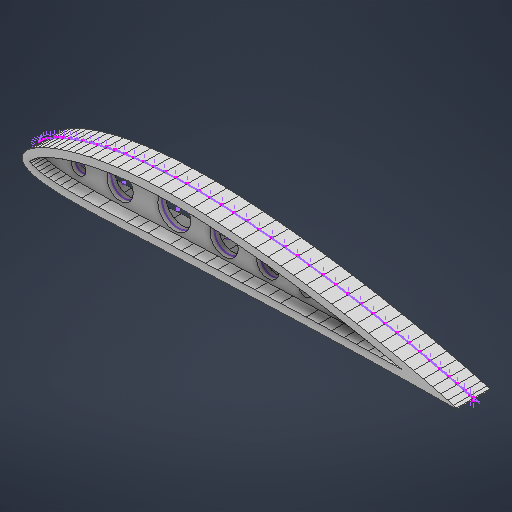
# Autodesk Inventor part: Profil NACA 4412
Saved by Autodesk Inventor 2026 (Build 300175050, 175E)
## iProperties
Created: 2026-01-17
Part Number: Profil NACA 4412
Material: Všeobecné
Document SubType Name: Modeling
Designer: marti
Density: 1 g/cm^3
Appearance: Výchozí
Author: marti
Autodesk Inventor part; units mm, degrees
ref_plane "YZ Plane" through (0, 0, 0) normal (1, 0, 0) x (0, 1, 0)
ref_plane "XZ Plane" through (0, 0, 0) normal (0, 1, 0) x (-1, 0, 0)
ref_plane "XY Plane" through (0, 0, 0) normal (0, 0, 1) x (1, 0, 0)
sketch "Náčrt1" plane through (-64.9965, -4.5129, 0) normal (0, 0, 1) x (1, 0, 0)
  line L0 (0, 0) -> (0.1008, -0.6172)
  line L1 (0.1008, -0.6172) -> (0.4005, -1.1751)
  line L2 (0.4005, -1.1751) -> (0.8948, -1.675)
  line L3 (0.8948, -1.675) -> (1.5794, -2.1181)
  line L4 (1.5794, -2.1181) -> (2.45, -2.5059)
  line L5 (2.45, -2.5059) -> (3.502, -2.8399)
  line L6 (3.502, -2.8399) -> (4.7309, -3.1217)
  line L7 (4.7309, -3.1217) -> (6.1321, -3.3532)
  line L8 (6.1321, -3.3532) -> (7.7009, -3.5364)
  line L9 (7.7009, -3.5364) -> (9.4326, -3.6734)
  line L10 (9.4326, -3.6734) -> (11.3221, -3.7667)
  line L11 (11.3221, -3.7667) -> (13.3646, -3.8188)
  line L12 (13.3646, -3.8188) -> (15.5549, -3.8188)
  line L13 (15.5549, -3.8188) -> (17.8877, -3.8188)
  line L14 (17.8877, -3.8188) -> (20.3578, -3.7585)
  line L15 (20.3578, -3.7585) -> (22.9603, -3.695)
  line L16 (22.9603, -3.695) -> (25.688, -3.5719)
  line L17 (25.688, -3.5719) -> (28.5365, -3.4433)
  line L18 (28.5365, -3.4433) -> (31.5001, -3.3096)
  line L19 (31.5001, -3.3096) -> (34.5717, -3.1509)
  line L20 (34.5717, -3.1509) -> (37.7458, -2.9903)
  line L21 (37.7458, -2.9903) -> (41.0158, -2.8272)
  line L22 (41.0158, -2.8272) -> (44.3749, -2.6597)
  line L23 (44.3749, -2.6597) -> (47.817, -2.512)
  line L24 (47.817, -2.512) -> (51.3342, -2.369)
  line L25 (51.3342, -2.369) -> (54.9194, -2.2327)
  line L26 (54.9194, -2.2327) -> (58.5651, -2.0885)
  line L27 (58.5651, -2.0885) -> (62.2634, -1.9385)
  line L28 (62.2634, -1.9385) -> (66.0059, -1.7856)
  line L29 (66.0059, -1.7856) -> (69.7841, -1.632)
  line L30 (69.7841, -1.632) -> (73.5888, -1.4803)
  line L31 (73.5888, -1.4803) -> (77.4106, -1.3325)
  line L32 (77.4106, -1.3325) -> (85.0644, -1.0556)
  line L33 (85.0644, -1.0556) -> (88.8745, -0.9296)
  line L34 (88.8745, -0.9296) -> (92.6573, -0.8132)
  line L35 (92.6573, -0.8132) -> (96.3998, -0.7072)
  line L36 (96.3998, -0.7072) -> (100.0878, -0.612)
  line L37 (100.0878, -0.612) -> (103.7057, -0.5276)
  line L38 (103.7057, -0.5276) -> (107.2363, -0.4539)
  line L39 (107.2363, -0.4539) -> (110.6603, -0.3905)
  line L40 (110.6603, -0.3905) -> (113.9558, -0.3368)
  line L41 (113.9558, -0.3368) -> (117.0974, -0.2918)
  line L42 (117.0974, -0.2918) -> (120.055, -0.2549)
  line L43 (120.055, -0.2549) -> (122.7911, -0.2251)
  line L44 (122.7911, -0.2251) -> (125.2574, -0.2014)
  line L45 (125.2574, -0.2014) -> (127.3856, -0.1834)
  line L46 (127.3856, -0.1834) -> (129.0641, -0.1691)
  line L47 (129.0641, -0.1691) -> (129.9931, -0.1612)
  line L48 (129.9931, -0.1612) -> (129.9906, 0.1321)
  line L49 (129.9906, 0.1321) -> (129.0576, 0.3875)
  line L50 (129.0576, 0.3875) -> (127.3795, 0.839)
  line L51 (127.3795, 0.839) -> (125.2516, 1.3993)
  line L52 (125.2516, 1.3993) -> (122.7858, 2.032)
  line L53 (122.7858, 2.032) -> (120.0501, 2.7132)
  line L54 (120.0501, 2.7132) -> (117.0931, 3.4254)
  line L55 (117.0931, 3.4254) -> (113.952, 4.1548)
  line L56 (113.952, 4.1548) -> (110.657, 4.8904)
  line L57 (110.657, 4.8904) -> (107.2335, 5.6228)
  line L58 (107.2335, 5.6228) -> (103.7034, 6.3444)
  line L59 (103.7034, 6.3444) -> (100.086, 7.0485)
  line L60 (100.086, 7.0485) -> (96.3985, 7.7294)
  line L61 (96.3985, 7.7294) -> (92.6565, 8.3822)
  line L62 (92.6565, 8.3822) -> (88.8741, 9.0026)
  line L63 (88.8741, 9.0026) -> (85.0644, 9.5868)
  line L64 (85.0644, 9.5868) -> (81.2394, 10.1289)
  line L65 (81.2394, 10.1289) -> (77.4106, 10.6287)
  line L66 (77.4106, 10.6287) -> (73.5888, 11.0836)
  line L67 (73.5888, 11.0836) -> (69.7841, 11.4914)
  line L68 (69.7841, 11.4914) -> (66.0059, 11.8502)
  line L69 (66.0059, 11.8502) -> (62.2634, 12.1585)
  line L70 (62.2634, 12.1585) -> (58.5651, 12.4148)
  line L71 (58.5651, 12.4148) -> (54.9194, 12.6181)
  line L72 (54.9194, 12.6181) -> (51.3342, 12.7673)
  line L73 (51.3342, 12.7673) -> (47.817, 12.8447)
  line L74 (47.817, 12.8447) -> (44.3752, 12.8426)
  line L75 (44.3752, 12.8426) -> (41.0158, 12.7632)
  line L76 (41.0158, 12.7632) -> (37.7458, 12.6088)
  line L77 (37.7458, 12.6088) -> (34.5717, 12.3826)
  line L78 (34.5717, 12.3826) -> (31.4999, 12.088)
  line L79 (31.4999, 12.088) -> (28.5366, 11.7287)
  line L80 (28.5366, 11.7287) -> (25.688, 11.3091)
  line L81 (25.688, 11.3091) -> (22.9598, 10.8338)
  line L82 (22.9598, 10.8338) -> (20.3578, 10.3077)
  line L83 (20.3578, 10.3077) -> (17.8877, 9.7359)
  line L84 (17.8877, 9.7359) -> (15.5548, 9.1241)
  line L85 (15.5548, 9.1241) -> (13.3646, 8.4777)
  line L86 (13.3646, 8.4777) -> (11.3221, 7.8025)
  line L87 (11.3221, 7.8025) -> (9.4326, 7.1042)
  line L88 (9.4326, 7.1042) -> (7.7009, 6.3887)
  line L89 (7.7009, 6.3887) -> (6.1321, 5.6614)
  line L90 (6.1321, 5.6614) -> (4.7309, 4.928)
  line L91 (4.7309, 4.928) -> (3.502, 4.1935)
  line L92 (3.502, 4.1935) -> (2.45, 3.4628)
  line L93 (2.45, 3.4628) -> (1.5794, 2.7403)
  line L94 (1.5794, 2.7403) -> (0.8948, 2.0298)
  line L95 (0.8948, 2.0298) -> (0.4005, 1.3347)
  line L96 (0.4005, 1.3347) -> (0.1008, 0.6574)
  line L97 (0.1008, 0.6574) -> (0, 0)
  point P0 (81.2394, -1.1904)
  constraints: 196 end point, 7 collinear, 2 perpendicular, 1 horizontal, 1 parallel
sketch "Náčrt2" plane through (0, 0, 0) normal (0, 0, 1) x (1, 0, 0)
  line L0 (-64.8957, -5.1301) -> (-64.596, -5.688) projected
  line L1 (-64.596, -5.688) -> (-64.1017, -6.1879) projected
  line L2 (-64.1017, -6.1879) -> (-63.4171, -6.631) projected
  line L3 (-63.4171, -6.631) -> (-62.5466, -7.0188) projected
  line L4 (-62.5466, -7.0188) -> (-61.4946, -7.3528) projected
  line L5 (-61.4946, -7.3528) -> (-60.2657, -7.6347) projected
  line L6 (-60.2657, -7.6347) -> (-58.8644, -7.8662) projected
  line L7 (-58.8644, -7.8662) -> (-57.2956, -8.0493) projected
  line L8 (-57.2956, -8.0493) -> (-55.564, -8.1863) projected
  line L9 (-55.564, -8.1863) -> (-53.6744, -8.2796) projected
  line L10 (-53.6744, -8.2796) -> (-51.632, -8.3318) projected
  line L11 (-51.632, -8.3318) -> (-47.1088, -8.3318) projected
  line L12 (-47.1088, -8.3318) -> (-42.0363, -8.208) projected
  line L13 (-42.0363, -8.208) -> (-33.4964, -7.8225) projected
  line L14 (-33.4964, -7.8225) -> (-30.4248, -7.6638) projected
  line L15 (-30.4248, -7.6638) -> (-27.2507, -7.5032) projected
  line L16 (-27.2507, -7.5032) -> (-20.6217, -7.1726) projected
  line L17 (-20.6217, -7.1726) -> (-17.1795, -7.0249) projected
  line L18 (-17.1795, -7.0249) -> (-13.6624, -6.882) projected
  line L19 (-13.6624, -6.882) -> (-10.0771, -6.7456) projected
  line L20 (-10.0771, -6.7456) -> (-6.4314, -6.6014) projected
  line L21 (-6.4314, -6.6014) -> (-2.7331, -6.4515) projected
  line L22 (-2.7331, -6.4515) -> (1.0094, -6.2985) projected
  line L23 (1.0094, -6.2985) -> (4.7875, -6.1449) projected
  line L24 (4.7875, -6.1449) -> (8.5923, -5.9932) projected
  line L25 (8.5923, -5.9932) -> (12.4141, -5.8454) projected
  line L26 (12.4141, -5.8454) -> (20.0679, -5.5686) projected
  line L27 (20.0679, -5.5686) -> (23.878, -5.4425) projected
  line L28 (23.878, -5.4425) -> (27.6608, -5.3262) projected
  line L29 (27.6608, -5.3262) -> (31.4033, -5.2202) projected
  line L30 (31.4033, -5.2202) -> (35.0913, -5.1249) projected
  line L31 (35.0913, -5.1249) -> (38.7092, -5.0406) projected
  line L32 (38.7092, -5.0406) -> (42.2397, -4.9669) projected
  line L33 (42.2397, -4.9669) -> (45.6637, -4.9035) projected
  line L34 (45.6637, -4.9035) -> (48.9593, -4.8497) projected
  line L35 (48.9593, -4.8497) -> (52.1009, -4.8048) projected
  line L36 (52.1009, -4.8048) -> (55.0584, -4.7678) projected
  line L37 (55.0584, -4.7678) -> (57.7946, -4.738) projected
  line L38 (57.7946, -4.738) -> (60.2609, -4.7144) projected
  line L39 (60.2609, -4.7144) -> (64.9965, -4.6742) projected
  line L40 (64.9965, -4.6742) -> (64.994, -4.3808) projected
  line L41 (64.994, -4.3808) -> (64.0611, -4.1254) projected
  line L42 (64.0611, -4.1254) -> (62.3829, -3.6739) projected
  line L43 (62.3829, -3.6739) -> (60.2551, -3.1136) projected
  line L44 (60.2551, -3.1136) -> (57.7893, -2.481) projected
  line L45 (57.7893, -2.481) -> (55.0536, -1.7998) projected
  line L46 (55.0536, -1.7998) -> (52.0966, -1.0876) projected
  line L47 (52.0966, -1.0876) -> (48.9554, -0.3581) projected
  line L48 (48.9554, -0.3581) -> (45.6604, 0.3774) projected
  line L49 (45.6604, 0.3774) -> (42.237, 1.1099) projected
  line L50 (42.237, 1.1099) -> (38.7069, 1.8315) projected
  line L51 (38.7069, 1.8315) -> (35.0895, 2.5356) projected
  line L52 (35.0895, 2.5356) -> (31.402, 3.2165) projected
  line L53 (31.402, 3.2165) -> (27.66, 3.8692) projected
  line L54 (27.66, 3.8692) -> (23.8776, 4.4896) projected
  line L55 (23.8776, 4.4896) -> (20.0679, 5.0739) projected
  line L56 (20.0679, 5.0739) -> (16.2428, 5.616) projected
  line L57 (16.2428, 5.616) -> (12.4141, 6.1158) projected
  line L58 (12.4141, 6.1158) -> (8.5923, 6.5707) projected
  line L59 (8.5923, 6.5707) -> (4.7875, 6.9785) projected
  line L60 (4.7875, 6.9785) -> (1.0094, 7.3373) projected
  line L61 (1.0094, 7.3373) -> (-2.7331, 7.6455) projected
  line L62 (-2.7331, 7.6455) -> (-6.4314, 7.9018) projected
  line L63 (-6.4314, 7.9018) -> (-10.0771, 8.1052) projected
  line L64 (-10.0771, 8.1052) -> (-13.6624, 8.2544) projected
  line L65 (-13.6624, 8.2544) -> (-17.1795, 8.3318) projected
  line L66 (-17.1795, 8.3318) -> (-20.6213, 8.3297) projected
  line L67 (-20.6213, 8.3297) -> (-23.9807, 8.2502) projected
  line L68 (-23.9807, 8.2502) -> (-27.2507, 8.0959) projected
  line L69 (-27.2507, 8.0959) -> (-30.4248, 7.8697) projected
  line L70 (-30.4248, 7.8697) -> (-33.4966, 7.575) projected
  line L71 (-33.4966, 7.575) -> (-36.4599, 7.2158) projected
  line L72 (-36.4599, 7.2158) -> (-39.3086, 6.7962) projected
  line L73 (-39.3086, 6.7962) -> (-42.0367, 6.3209) projected
  line L74 (-42.0367, 6.3209) -> (-44.6387, 5.7947) projected
  line L75 (-44.6387, 5.7947) -> (-47.1088, 5.223) projected
  line L76 (-47.1088, 5.223) -> (-49.4417, 4.6111) projected
  line L77 (-49.4417, 4.6111) -> (-51.632, 3.9647) projected
  line L78 (-51.632, 3.9647) -> (-53.6744, 3.2895) projected
  line L79 (-53.6744, 3.2895) -> (-55.564, 2.5913) projected
  line L80 (-55.564, 2.5913) -> (-57.2956, 1.8757) projected
  line L81 (-57.2956, 1.8757) -> (-58.8644, 1.1485) projected
  line L82 (-58.8644, 1.1485) -> (-60.2657, 0.4151) projected
  line L83 (-60.2657, 0.4151) -> (-61.4946, -0.3194) projected
  line L84 (-61.4946, -0.3194) -> (-62.5466, -1.0501) projected
  line L85 (-62.5466, -1.0501) -> (-63.4171, -1.7727) projected
  line L86 (-63.4171, -1.7727) -> (-64.1017, -2.4831) projected
  line L87 (-64.1017, -2.4831) -> (-64.596, -3.1783) projected
  line L88 (-64.596, -3.1783) -> (-64.8957, -3.8555) projected
  line L89 (-64.8957, -3.8555) -> (-64.9965, -4.5129) projected
  line L90 (-64.9965, -4.5129) -> (-64.8957, -5.1301) projected
  line L91 (-44.1584, 3.5791) -> (-41.6175, 4.0929)
  line L92 (-41.6175, 4.0929) -> (-38.9488, 4.5579)
  line L93 (-38.9488, 4.5579) -> (-36.1583, 4.9689)
  line L94 (-36.1583, 4.9689) -> (-33.252, 5.3212)
  line L95 (-33.252, 5.3212) -> (-30.236, 5.6105)
  line L96 (-30.236, 5.6105) -> (-27.1167, 5.8328)
  line L97 (-27.1167, 5.8328) -> (-23.9004, 5.9846)
  line L98 (-23.9004, 5.9846) -> (-20.5938, 6.0628)
  line L99 (-20.5938, 6.0628) -> (-17.2038, 6.0649)
  line L100 (-17.2038, 6.0649) -> (-13.7344, 5.9886)
  line L101 (-13.7344, 5.9886) -> (-10.1874, 5.841)
  line L102 (-10.1874, 5.841) -> (-6.5729, 5.6393)
  line L103 (-6.5729, 5.6393) -> (-2.9045, 5.3851)
  line L104 (-2.9045, 5.3851) -> (0.8092, 5.0792)
  line L105 (0.8092, 5.0792) -> (4.5596, 4.7231)
  line L106 (4.5596, 4.7231) -> (8.3375, 4.3181)
  line L107 (8.3375, 4.3181) -> (12.1334, 3.8663)
  line L108 (12.1334, 3.8663) -> (15.9371, 3.3698)
  line L109 (15.9371, 3.3698) -> (19.737, 2.8313)
  line L110 (19.737, 2.8313) -> (23.5223, 2.2507)
  line L111 (23.5223, 2.2507) -> (27.2817, 1.6341)
  line L112 (27.2817, 1.6341) -> (31.0014, 0.9852)
  line L113 (31.0014, 0.9852) -> (34.6671, 0.3084)
  line L114 (34.6671, 0.3084) -> (38.2634, -0.3916)
  line L115 (38.2634, -0.3916) -> (41.7728, -1.109)
  line L116 (41.7728, -1.109) -> (45.1763, -1.8372)
  line L117 (45.1763, -1.8372) -> (48.4521, -2.5684)
  line L118 (48.4521, -2.5684) -> (48.542, -2.5893)
  line L119 (48.542, -2.5893) -> (45.6243, -2.6369)
  line L120 (45.6243, -2.6369) -> (42.1951, -2.7005)
  line L121 (42.1951, -2.7005) -> (38.6591, -2.7742)
  line L122 (38.6591, -2.7742) -> (35.0356, -2.8587)
  line L123 (35.0356, -2.8587) -> (31.342, -2.9541)
  line L124 (31.342, -2.9541) -> (27.5939, -3.0603)
  line L125 (27.5939, -3.0603) -> (23.8056, -3.1768)
  line L126 (23.8056, -3.1768) -> (19.9895, -3.3031)
  line L127 (19.9895, -3.3031) -> (12.3293, -3.5801)
  line L128 (12.3293, -3.5801) -> (8.5033, -3.7281)
  line L129 (8.5033, -3.7281) -> (4.6964, -3.8799)
  line L130 (4.6964, -3.8799) -> (0.9171, -4.0335)
  line L131 (0.9171, -4.0335) -> (-2.8253, -4.1865)
  line L132 (-2.8253, -4.1865) -> (-6.5221, -4.3363)
  line L133 (-6.5221, -4.3363) -> (-10.165, -4.4805)
  line L134 (-10.165, -4.4805) -> (-13.7515, -4.6169)
  line L135 (-13.7515, -4.6169) -> (-17.2742, -4.76)
  line L136 (-17.2742, -4.76) -> (-20.7267, -4.9082)
  line L137 (-20.7267, -4.9082) -> (-27.3644, -5.2392)
  line L138 (-27.3644, -5.2392) -> (-30.5406, -5.3999)
  line L139 (-30.5406, -5.3999) -> (-33.606, -5.5583)
  line L140 (-33.606, -5.5583) -> (-42.115, -5.9423)
  line L141 (-42.115, -5.9423) -> (-47.1365, -6.0649)
  line L142 (-47.1365, -6.0649) -> (-51.603, -6.0649)
  line L143 (-51.603, -6.0649) -> (-53.5896, -6.0142)
  line L144 (-53.5896, -6.0142) -> (-55.4186, -5.9239)
  line L145 (-55.4186, -5.9239) -> (-57.0747, -5.7928)
  line L146 (-57.0747, -5.7928) -> (-58.5481, -5.6208)
  line L147 (-58.5481, -5.6208) -> (-59.8271, -5.4095)
  line L148 (-59.8271, -5.4095) -> (-60.8972, -5.1641)
  line L149 (-60.8972, -5.1641) -> (-61.7399, -4.8966)
  line L150 (-61.7399, -4.8966) -> (-62.3335, -4.6322)
  line L151 (-62.3335, -4.6322) -> (-62.6631, -4.4188)
  line L152 (-62.6631, -4.4188) -> (-62.6651, -4.4167)
  line L153 (-62.6651, -4.4167) -> (-62.6158, -4.3052)
  line L154 (-62.6158, -4.3052) -> (-62.3522, -3.9344)
  line L155 (-62.3522, -3.9344) -> (-61.8723, -3.4364)
  line L156 (-61.8723, -3.4364) -> (-61.1736, -2.8565)
  line L157 (-61.1736, -2.8565) -> (-60.2651, -2.2255)
  line L158 (-60.2651, -2.2255) -> (-59.1577, -1.5636)
  line L159 (-59.1577, -1.5636) -> (-57.8615, -0.8852)
  line L160 (-57.8615, -0.8852) -> (-56.3857, -0.2011)
  line L161 (-56.3857, -0.2011) -> (-54.7379, 0.4798)
  line L162 (-54.7379, 0.4798) -> (-52.9256, 1.1496)
  line L163 (-52.9256, 1.1496) -> (-50.9552, 1.8009)
  line L164 (-50.9552, 1.8009) -> (-48.8332, 2.4272)
  line L165 (-48.8332, 2.4272) -> (-46.5656, 3.0219)
  line L166 (-46.5656, 3.0219) -> (-44.1584, 3.5791)
  circle A0 centre (-39.3753, -0.8852) radius 3.9303
  circle A1 centre (-23.1981, 0.4798) radius 4.9194
  circle A2 centre (-8.2542, 0.4798) radius 4.211
  circle A3 centre (4.7875, 0.4798) radius 3.3527
  circle A4 centre (-51.8098, -2.2255) radius 2.1974
  circle A5 centre (16.0359, -0.0281) radius 2.0007
  point P0 (0, 0)
  constraints: 152 end point, 6 centre point, 75 other
extrude "Vysunutí2" add sketch "Náčrt2" along normal mid plane 10 contours L90 L89 L88 L87 L86 L85 L84 L83 L82 L81 L80 L79 L78 L77 L76 L75 L74 L73 L72 L71 L70 L69 L68 L67 L66 L65 L64 L63 L62 L61 L60 L59 L58 L57 L56 L55 L54 L53 L52 L51 L50 L49 L48 L47 L46 L45 L44 L43 L42 L41 L40 L39 L38 L37 L36 L35 L34 L33 L32 L31 L30 L29 L28 L27 L26 L25 L24 L23 L22 L21 L20 L19 L18 L17 L16 L15 L14 L13 L12 L11 L10 L9 L8 L7 L6 L5 L4 L3 L2 L1 L0
extrude "Vysunutí3" add sketch "Náčrt2" along normal mid plane 2.5 contours L91 L92 L93 L94 L95 L96 L97 L98 L99 L100 L101 L102 L103 L104 L105 L106 L107 L108 L109 L110 L111 L112 L113 L114 L115 L116 L117 L118 L119 L120 L121 L122 L123 L124 L125 L126 L127 L128 L129 L130 L131 L132 L133 L134 L135 L136 L137 L138 L139 L140 L141 L142 L143 L144 L145 L146 L147 L148 L149 L150 L151 L152 L153 L154 L155 L156 L157 L158 L159 L160 L161 L162 L163 L164 L165 L166
